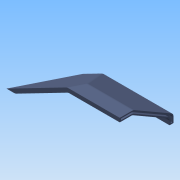
# Autodesk Inventor part: термокрышка
Saved by Autodesk Inventor 2017 (Build 210142000, 142)
## iProperties
Part Number: термокрышка
Material: Типовые
Document SubType Name: Modeling
Designer: Max
Density: 1 g/cm^3
Appearance: Резина — синяя
Mass: 49.5484 g
Surface Area: 232.53 cm^2
Volume: 49.5484 cm^3
Author: Max
Autodesk Inventor part; units mm, degrees
ref_plane "YZ Plane" through (0, 0, 0) normal (1, 0, 0) x (0, 1, 0)
ref_plane "XZ Plane" through (0, 0, 0) normal (0, 1, 0) x (-1, 0, 0)
ref_plane "XY Plane" through (0, 0, 0) normal (0, 0, 1) x (1, 0, 0)
sketch "Эскиз2" plane through (0, 0, 0) normal (0, 0, 1) x (1, 0, 0)
  circle A0 centre (181, -158) radius 2 projected
  circle A1 centre (-181, 158) radius 2 projected
  circle A2 centre (181, 158) radius 2 projected
  circle A3 centre (-181, -158) radius 2 projected
  circle A4 centre (15.5, 126.5) radius 1.5 projected
  circle A5 centre (-15.5, 157.5) radius 1.5 projected
  circle A6 centre (15.5, 157.5) radius 1.5 projected
  circle A7 centre (-15.5, 126.5) radius 1.5 projected
  line L0 (89, 108) -> (89, 96) projected
  line L1 (89, 96) -> (69, 96) projected
  line L2 (69, 96) -> (69, 108) projected
  line L3 (69, 108) -> (89, 108) projected
  line L4 (168.6, 126.6) -> (168.6, 100.6) projected
  line L5 (168.6, 100.6) -> (140.6, 100.6) projected
  line L6 (140.6, 100.6) -> (140.6, 126.6) projected
  line L7 (140.6, 126.6) -> (168.6, 126.6) projected
  circle A8 centre (-92.5, 142) radius 6 projected
  circle A9 centre (-103.5, 142) radius 1.5 projected
  circle A10 centre (103.5, 142) radius 1.5 projected
  circle A11 centre (81.5, 142) radius 1.5 projected
  circle A12 centre (-81.5, 142) radius 1.5 projected
  circle A13 centre (92.5, 142) radius 6 projected
  circle A14 centre (0, 142) radius 11.5 projected
  line L8 (-107.3915, -104.3944) -> (-139.1034, -168)
  line L9 (107.3915, -104.3944) -> (-107.3915, -104.3944) projected
  line L10 (139.1034, -168) -> (107.3915, -104.3944)
  line L11 (189, 166) -> (189, -166) projected
  line L12 (-189, 166) -> (189, 166) projected
  line L13 (-189, -166) -> (-189, 166) projected
  line L14 (189, -168) -> (-189, -168) projected
  line L15 (-184, -161) -> (-184, 161)
  line L16 (-184, 161) -> (184, 161)
  line L17 (184, 161) -> (184, -161)
  line L18 (144.6904, -168) -> (110.4856, -99.3944)
  line L19 (110.4856, -99.3944) -> (-110.4856, -99.3944)
  line L20 (-110.4856, -99.3944) -> (-144.6904, -168)
  line L21 (-144.6904, -168) -> (144.6904, -168)
  point P0 (0, 0)
  dimension "d9" = 5
  constraints: 18 end point, 4 point on line, 1 collinear, 2 other
  measures "d9" distance between parallel lines of L8 L20
extrude "Выдавливание1" add sketch "Эскиз2" along normal blind 50 contours L9 L10 L14 L8 | L8 L14 L20 L19 L18 L10 L9
sketch "Эскиз4" plane through (-144.6904, -168, 0) normal (0, -1, 0) x (1, 0, 0)
  line L0 (59.1192, 66.315) -> (219.6093, 66.315)
  line L1 (219.6093, 66.315) -> (219.6093, 40)
  line L2 (219.6093, 40) -> (59.1192, 40)
  line L3 (59.1192, 40) -> (59.1192, 66.315)
  line L4 (0, 0) -> (289.3807, 0) projected
  point P0 (144.6904, 0)
  dimension "d20" = 40
  constraints: 8 end point, 2 parallel, 1 horizontal, 1 perpendicular
  measures "d20" distance between parallel lines of L4 L2
draft "НаклГрань6" angle 30 pull direction (0, 1, 0) faces at (36.8285, -145.1315, 50) fixed edges at (0, -168, 50)
draft "НаклГрань7" angle 60 pull direction (0, 0, 1) faces at (133.2888, -145.1315, 20.1302) fixed edges at (127.588, -133.6972, 0)
draft "НаклГрань8" angle 60 pull direction (0, 0, 1) faces at (-133.2888, -145.1315, 20.1302) fixed edges at (-127.588, -133.6972, 0)
extrude "Выдавливание3" cut sketch "Эскиз4" against normal blind 60
shell "Оболочка1" thickness 5 removed faces 2 at (-22.425, -168, 13.3333) at (36.8285, -145.1315, 0)
fillet "Сопряжение1" radius 5 2 edges at (-117.6605, -136.1972, 0) (117.6605, -136.1972, 0)
fillet "Сопряжение2" radius 5 9 edges at (-72.5461, -128.2068, 21.2519) (-101.8555, -104.3944, 0.1704) (-93.8949, -104.3944, 4.0868) (0, -104.3944, 7.5038) (0, -152.0192, 35) (-61.7941, -160.0096, 35) (61.7941, -160.0096, 35) (72.5461, -128.2068, 21.2519) (93.8949, -104.3944, 4.0868)
fillet "Сопряжение3" radius 5 8 edges at (62.9572, -159.3397, 40) (-62.9572, -159.3397, 40) (0, -150.6795, 40) (-74.5077, -125.037, 25.1953) (74.5077, -125.037, 25.1953) (100.4308, -99.3944, 5.1953) (0, -99.3944, 10.3906) (-100.4308, -99.3944, 5.1953)
sketch "Эскиз6" plane through (-144.6904, -168, 0) normal (0, -1, 0) x (1, 0, 0)
  line L0 (-18.9062, 116.0026) -> (144.6904, 116.0026)
  line L1 (144.6904, 116.0026) -> (144.6904, -65.2449)
  line L2 (144.6904, -65.2449) -> (-18.9062, -65.2449)
  line L3 (-18.9062, -65.2449) -> (-18.9062, 116.0026)
  line L4 (144.6904, 116.0026) -> (305.7421, 116.0026)
  line L5 (305.7421, 116.0026) -> (305.7421, -65.2449)
  line L6 (305.7421, -65.2449) -> (144.6904, -65.2449)
  line L7 (144.6904, -65.2449) -> (144.6904, 116.0026)
  line L8 (279.7038, 0) -> (289.3807, 0) projected
  point P0 (144.6904, 0)
  point P1 (0, 0)
  dimension "d38" = 144.6904
  dimension "d39" = 144.6904
  constraints: 16 end point, 4 parallel, 2 horizontal, 2 perpendicular, 1 point on line
  measures "d38" distance from line of L1 L8.end
  measures "d39" distance from line of point (0, 0) L1
extrude "Выдавливание4" cut sketch "Эскиз6" against normal blind 200 contours L4 L5 L6 L1
sketch "Эскиз7" plane through (0, -168, 40) normal (1, 0, 0) x (0, 0, -1)
  line L0 (0, 0) -> (0, 15.9808) projected
  line L1 (5, 0) -> (0, 0) projected
  line L2 (5, 14.641) -> (5, 0) projected
  arc A0 (5.6699, 17.141) -> (5, 14.641) centre (10, 14.641) ccw projected
  line L3 (31.0528, 61.1056) -> (5.6699, 17.141) projected
  arc A1 (35.3829, 63.6056) -> (31.0528, 61.1056) centre (35.3829, 58.6056) ccw projected
  line L4 (40, 63.6056) -> (35.3829, 63.6056) projected
  line L5 (40, 68.6056) -> (40, 63.6056) projected
  line L6 (32.4962, 68.6056) -> (40, 68.6056) projected
  arc A2 (32.4962, 68.6056) -> (28.1661, 66.1056) centre (32.4962, 63.6056) ccw projected
  line L7 (0.6699, 18.4808) -> (28.1661, 66.1056) projected
  arc A3 (0.6699, 18.4808) -> (0, 15.9808) centre (5, 15.9808) ccw projected
  arc A4 (32.4962, 67.1056) -> (29.4651, 65.3556) centre (32.4962, 63.6056) ccw
  line L8 (32.4962, 67.1056) -> (38.5, 67.1056)
  line L9 (38.5, 67.1056) -> (38.5, 65.1056)
  line L10 (38.5, 65.1056) -> (35.3829, 65.1056)
  arc A5 (35.3829, 65.1056) -> (29.7538, 61.8556) centre (35.3829, 58.6056) ccw
  line L11 (29.7538, 61.8556) -> (4.3708, 17.891)
  arc A6 (4.3708, 17.891) -> (3.5, 14.641) centre (10, 14.641) ccw
  line L12 (3.5, 14.641) -> (3.5, 1.5)
  line L13 (3.5, 1.5) -> (1.5, 1.5)
  line L14 (1.5, 1.5) -> (1.5, 15.9808)
  arc A7 (1.9689, 17.7308) -> (1.5, 15.9808) centre (5, 15.9808) ccw
  line L15 (1.9689, 17.7308) -> (29.4651, 65.3556)
  point P0 (40, 168)
  dimension "d42" = 1.5
  constraints: 16 end point, 8 point on circle, 4 centre point, 11 other
  measures "d42" distance between parallel lines of L7 L15
extrude "Выдавливание5" cut sketch "Эскиз7" against normal blind 5 contours L8 L9 L10 A5 L11 A6 L12 L13 L14 A7 L15 A4
